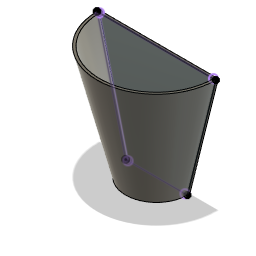
Checker Feeeder v1 (Autodesk Fusion 360 design; units mm, degrees)
Autodesk Fusion 360 part; units mm, degrees
sketch "Sketch1" plane through (0, 0, 0) normal (0, 0, 1) x (1, 0, 0)
  line L0 (0, 0) -> (38.1, 0) construction
  line L1 (0, 0) -> (0, 152.4) construction
  line L2 (0, 152.4) -> (76.2, 152.4) construction
  line L3 (76.2, 152.4) -> (38.1, 0)
  line L4 (79.4727, 152.4) -> (41.3727, 0)
  line L5 (38.1, 0) -> (41.3727, 0)
  line L6 (76.2, 152.4) -> (79.4727, 152.4)
  dimension "d1" = 38.1
  dimension "d2" = 152.4
  dimension "d3" = 76.2
  constraint coincident L0.start L1.start
  constraint horizontal L0
  constraint perpendicular L0 L1
  constraint perpendicular L1 L2
  constraint parallel L0 L5
  constraint parallel L3 L4
  constraint parallel L2 L6
  measures "d1" distance of L0.start L0.end
  measures "d2" distance of L0.start L1.end
  measures "d3" distance of L1.end L2.end
revolve "Revolve1" add sketch "Sketch1" angle 180 about axis through (0, 0, 0) along (0, -1, 0)
sketch "Sketch2" plane through (0, 0, 0) normal (0, 0, -1) x (-1, 0, 0)
  line L0 (-41.3727, 0) -> (-38.1, 0)
  line L1 (-38.1, 0) -> (-76.2, 152.4)
  line L2 (-76.2, 152.4) -> (-79.4727, 152.4)
  line L3 (-79.4727, 152.4) -> (-41.3727, 0)
  line L4 (38.1, 0) -> (41.3727, 0)
  line L5 (41.3727, 0) -> (79.4727, 152.4)
  line L6 (79.4727, 152.4) -> (76.2, 152.4)
  line L7 (76.2, 152.4) -> (38.1, 0)
  line L8 (-76.2, 152.4) -> (76.2, 152.4)
  line L9 (-38.1, 0) -> (38.1, 0)
  line L10 (-79.4727, 152.4) -> (79.4727, 152.4)
  line L11 (-41.3727, 0) -> (41.3727, 0)
  line L12 (79.4727, 152.4) -> (41.3727, 0)
  line L13 (-79.4727, 152.4) -> (-41.3727, 0)
  constraint coincident L2.end L3.start
  constraint coincident L5.end L6.start
  constraint coincident L0.start L3.end
  constraint coincident L4.end L5.start
extrude "Extrude2" add sketch "Sketch2" along normal blind 3.175
equation "d1 = ( 3 / 2 ) * 1 in"
